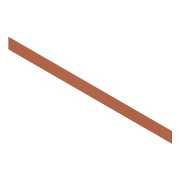
# Autodesk Inventor part: rf transmission plate
Saved by Autodesk Inventor 2011 (Build 150239000, 239)
## iProperties
Created: 2011-06-08
Part Number: rf transmission plate
Document SubType Name: Modeling
Designer: ijs09
Density: 1 g/cm^3
Author: ijs09
Autodesk Inventor part; units mm, degrees
ref_plane "YZ Plane" through (0, 0, 0) normal (1, 0, 0) x (0, 1, 0)
ref_plane "XZ Plane" through (0, 0, 0) normal (0, 1, 0) x (-1, 0, 0)
ref_plane "XY Plane" through (0, 0, 0) normal (0, 0, 1) x (1, 0, 0)
sketch "Sketch2" plane through (0, 0, 0) normal (0, 1, 0) x (-1, 0, 0)
  line L0 (-425, 28) -> (425, 28)
  line L1 (425, 28) -> (425, -28)
  line L2 (425, -28) -> (-425, -28)
  line L3 (-425, -28) -> (-425, 28)
  point P0 (0, 0)
  dimension "d0" = 56
  dimension "d1" = 28
  dimension "d2" = 850
  dimension "d3" = 425
  constraints: 8 end point, 2 parallel, 1 horizontal, 1 perpendicular
  measures "d0" distance between parallel lines of L0 L2
  measures "d1" distance from line of point (0, 0) L0
  measures "d2" distance between parallel lines of L3 L1
  measures "d3" distance from line of point (0, 0) L3
extrude "Extrusion1" add sketch "Sketch2" along normal blind 2
equation "\"d1\" = 0.5 * d0"
equation "\"d3\" = 0.5 * d2"
body "Solid1"
